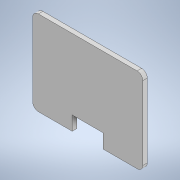
# Autodesk Inventor part: pcb_balun_top
Saved by Autodesk Inventor 2020.2 (Build 242310000, 310)
## iProperties
Created: 2020-09-26
Part Number: pcb_balun_top
Material: Generic
Document SubType Name: Modeling
Designer: Krishna Makhija
Density: 1 g/cm^3
Appearance: Default
Author: Krishna Makhija
Autodesk Inventor part; units mm, degrees
ref_plane "YZ Plane" through (0, 0, 0) normal (1, 0, 0) x (0, 1, 0)
ref_plane "XZ Plane" through (0, 0, 0) normal (0, 1, 0) x (-1, 0, 0)
ref_plane "XY Plane" through (0, 0, 0) normal (0, 0, 1) x (1, 0, 0)
sketch "Sketch2" plane through (0, 0, 0) normal (0, 0, 1) x (1, 0, 0)
  line L0 (-19.4999, -12.4999) -> (-19.4999, 12.4999)
  line L1 (-19.4999, 12.4999) -> (19.4999, 12.4999)
  line L2 (19.4999, 12.4999) -> (19.4999, -12.4999)
  line L3 (19.4999, -12.4999) -> (-19.4999, 12.4999) construction
  line L4 (-19.4999, -12.4999) -> (19.4999, 12.4999) construction
  line L5 (-5.4999, -12.4999) -> (-5.4999, -17.4996)
  line L6 (-5.4999, -17.4996) -> (-19.4999, -17.4996)
  line L7 (-19.4999, -17.4996) -> (-19.4999, -12.4999)
  line L8 (5.4995, -12.4999) -> (5.4995, -17.4996)
  line L9 (5.4995, -17.4996) -> (19.4999, -17.4996)
  line L10 (19.4999, -17.4996) -> (19.4999, -12.4999)
  line L11 (-5.4999, -12.4999) -> (5.4995, -12.4999)
  point P0 (0, 0)
  constraints: 24 end point, 3 parallel, 2 midpoint, 1 horizontal, 1 point on line
extrude "Extrusion2" add sketch "Sketch2" along normal blind 1.6
fillet "Fillet3" radius 2 4 edges at (19.4999, 12.4999, 0.8) (-19.4999, 12.4999, 0.8) (19.4999, -17.4996, 0.8) (-19.4999, -17.4996, 0.8)
body "Solid2"
